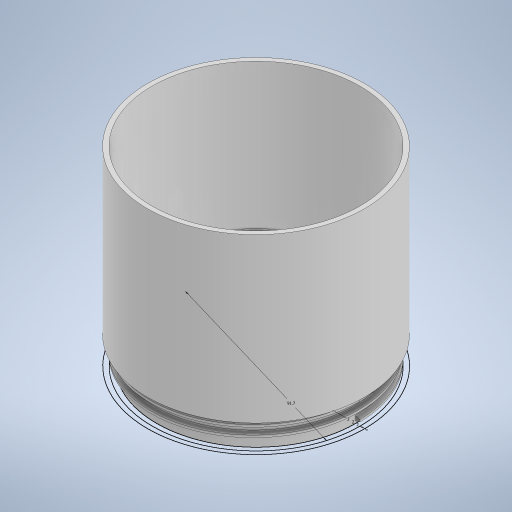
# Autodesk Inventor part: 탄두옆면2
Saved by Autodesk Inventor 2023 (Build 270158000, 158)
## iProperties
Created: 2023-10-31
Part Number: 탄두옆면2
Material: 일반
Document SubType Name: Modeling
Designer: rlatk
Density: 1 g/cm^3
Appearance: 기본값
Author: rlatk
Autodesk Inventor part; units mm, degrees
ref_plane "YZ Plane" through (0, 0, 0) normal (1, 0, 0) x (0, 1, 0)
ref_plane "XZ Plane" through (0, 0, 0) normal (0, 1, 0) x (-1, 0, 0)
ref_plane "XY Plane" through (0, 0, 0) normal (0, 0, 1) x (1, 0, 0)
sketch "스케치1" plane through (0, 0, 0) normal (0, 1, 0) x (-1, 0, 0)
  circle A0 centre (0, 0) radius 45.85
  circle A1 centre (0, 0) radius 47.85
  circle A2 centre (0, 0) radius 43.85
  circle A3 centre (0, 0) radius 41.85
  dimension "d0" = 91.7
  dimension "d1" = 2
  dimension "d22" = 2
  dimension "d23" = 2
  constraints: 4 centre point, 1 coincident
  measures "d0" diameter of A0
  measures "d1" radial gap between concentric circles of A0 A1
  measures "d22" radial gap between concentric circles of A0 A2
  measures "d23" radial gap between concentric circles of A2 A3
extrude "돌출1" add sketch "스케치1" along normal blind 84 contours A1
extrude "돌출4" add sketch "스케치1" along normal blind 20 contours A0 | A2
extrude "돌출5" cut sketch "스케치1" along normal blind 12 contours A0 | A1
sketch "스케치3" plane through (0, 0, 0) normal (0, 0, 1) x (1, 0, 0)
  line L0 (43.85, 12) -> (43.85, 0) projected
  line L1 (43.85, 1) -> (45.85, 1)
  line L2 (45.85, 1) -> (45.85, 3)
  line L3 (45.85, 3) -> (43.85, 3)
  line L4 (43.85, 3) -> (43.85, 1)
  line L5 (43.85, 1) -> (45.85, 1.5)
  line L6 (45.85, 2.5) -> (43.85, 3)
  point P0 (0, 0)
  dimension "d28" = 2
  dimension "d29" = 2
  dimension "d30" = 1
  dimension "d31" = 0.5
  dimension "d32" = 0.5
  constraints: 12 end point, 3 point on line, 2 parallel, 1 horizontal, 1 perpendicular
  measures "d28" distance of L3.end L2.end
  measures "d29" distance of L2.end L1.end
  measures "d30" distance of L1.start L0.end
  measures "d31" distance of L2.end L6.start
  measures "d32" distance of L5.end L1.end
coil "코일2" sketch "스케치3" operation add axis through (0, -10, 0) along (0, 1, 0) pitch 4 turns 2 hand right contours L6 L2 L5 L0
